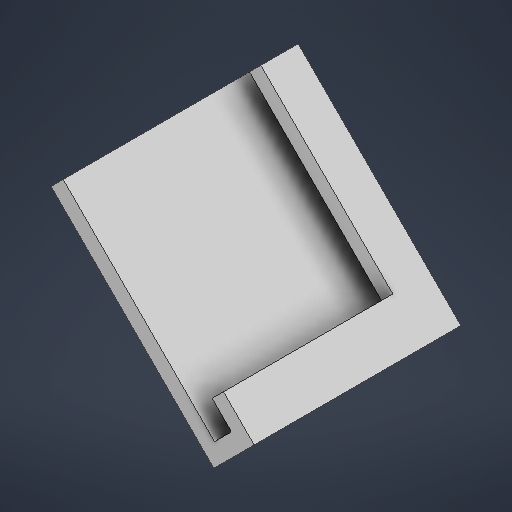
# Autodesk Inventor part: фанера
Saved by Autodesk Inventor 2025 (Build 290162000, 162)
## iProperties
Created: 2025-01-09
Part Number: фанера
Material: Типовые
Document SubType Name: Modeling
Designer: Phantom
Density: 1 g/cm^3
Appearance: По умолчанию
Author: Phantom
Autodesk Inventor part; units mm, degrees
ref_plane "YZ Plane" through (0, 0, 0) normal (1, 0, 0) x (0, 1, 0)
ref_plane "XZ Plane" through (0, 0, 0) normal (0, 1, 0) x (-1, 0, 0)
ref_plane "XY Plane" through (0, 0, 0) normal (0, 0, 1) x (1, 0, 0)
sketch "Эскиз1" plane through (0, 0, 0) normal (0, 0, 1) x (1, 0, 0)
  line L0 (0, 80) -> (80, 0)
  line L1 (2.2627, 82.2627) -> (82.2627, 2.2627)
  line L2 (0, 80) -> (2.2627, 82.2627)
  line L3 (80, 0) -> (82.2627, 2.2627)
  point P0 (0, 0)
  dimension "d2" = 3.2
  constraints: 8 end point, 2 perpendicular, 1 parallel
  measures "d2" distance between parallel lines of L0 L1
extrude "Выдавливание1" add sketch "Эскиз1" along normal blind 38.75
sketch "Эскиз2" plane through (0, 0, 0) normal (0, 0, -1) x (-1, 0, 0)
  line L0 (0, 80) -> (-80, 0) projected
  line L1 (-55, 25) -> (-55, -25)
  line L2 (-80, 0) -> (-55, 0)
  line L3 (-55, 8) -> (-60, 8)
  line L4 (-60, 8) -> (-60, 33)
  circle A0 centre (-60, 12) radius 2
  circle A1 centre (-60, 5) radius 2
  point P0 (0, 0)
  dimension "d5" = 4
  constraints: 8 end point, 3 point on line, 2 centre point, 1 horizontal, 1 midpoint, 1 perpendicular, 1 vertical
  measures "d5" diameter of A0
extrude "Выдавливание2" add sketch "Эскиз2" against normal blind 3 contours L1 L3 L4 A0 L0 | L4 A0 L3 L1 L2 L0
sketch "Эскиз3" plane through (2.2627, 82.2627, 0) normal (0.7071068, 0.7071068, 0) x (-0.7071068, 0.7071068, 0)
  line L0 (-113.1371, 0) -> (-95.4594, 0) projected
  line L1 (0, 38.75) -> (-113.1371, 38.75) projected
  line L2 (-113.1371, 0) -> (-110.1371, 0)
  line L3 (-110.1371, 0) -> (-110.1371, 38.75)
  line L4 (-110.1371, 38.75) -> (-113.1371, 38.75)
  line L5 (-113.1371, 38.75) -> (-113.1371, 0)
  point P0 (-56.5685, 0)
  point P1 (-113.1371, 38.75)
  dimension "d8" = 3
  constraints: 8 end point, 2 parallel, 1 horizontal, 1 perpendicular, 1 point on line
  measures "d8" distance of L4.end L3.end
extrude "Выдавливание3" add sketch "Эскиз3" along normal blind 4.5
sketch "Эскиз4" plane through (5.4447, 85.4447, 0) normal (0.7071068, 0.7071068, 0) x (0, 0, 1)
  line L0 (0, 113.1371) -> (3, 113.1371) projected
  line L1 (0, 0) -> (38.75, 0) projected
  line L2 (0, 113.1371) -> (7, 113.1371)
  line L3 (7, 113.1371) -> (7, 0)
  line L4 (7, 0) -> (0, 0)
  line L5 (0, 0) -> (0, 113.1371)
  line L6 (38.75, 0) -> (38.75, 113.1371) projected
  line L7 (7, 113.1371) -> (38.75, 113.1371)
  line L8 (38.75, 113.1371) -> (38.75, 105)
  line L9 (38.75, 105) -> (7, 105)
  line L10 (7, 105) -> (7, 113.1371)
  point P0 (0, 56.5685)
  point P1 (38.75, 113.1371)
  point P2 (7, 105)
  constraints: 16 end point, 4 parallel, 2 horizontal, 2 perpendicular, 2 point on line
extrude "Выдавливание4" add sketch "Эскиз4" along normal blind 3 contours L0 L2 L3 L1 L5 | L7 L6 L9 L3
sketch "Эскиз5" plane through (0, 0, 0) normal (0, 0, -1) x (-1, 0, 0)
  line L0 (-80.1414, 4.3841) -> (-2.2627, 82.2627) projected
  circle A0 centre (-60, 12) radius 2 projected
  circle A1 centre (-60, 5) radius 2 projected
  line L1 (0, 80) -> (-55, 25) projected
  line L2 (-2.2627, 82.2627) -> (0, 80) projected
  line L3 (-80.1414, 4.3841) -> (-2.2627, 82.2627) projected
  line L4 (-80.1414, 4.3841) -> (-83.3234, 7.566) projected
  line L5 (-83.3234, 7.566) -> (-5.4447, 85.4447) projected
  line L6 (-5.4447, 85.4447) -> (-7.566, 87.566) projected
  line L7 (-87.566, 7.566) -> (-7.566, 87.566) projected
  line L8 (-80, 0) -> (-87.566, 7.566) projected
  line L9 (-80, 0) -> (-55, 0) projected
  line L10 (-55, 0) -> (-55, 25) projected
  line L11 (-5.4447, 85.4447) -> (-2.2627, 82.2627)
  line L12 (-83.3234, 7.566) -> (-5.4447, 85.4447) projected
  point P0 (0, 0)
  point P1 (-2.2627, 82.2627)
  constraints: 2 end point, 1 perpendicular
extrude "Выдавливание5" add sketch "Эскиз5" against normal blind 3 contours L4 L5 L11 L0
sketch "Эскиз6" plane through (7.566, 87.566, 0) normal (0.7071068, 0.7071068, 0) x (-0.7071068, 0.7071068, 0)
  line L0 (0, 0) -> (-77.7817, 0) projected
  line L1 (-110.1371, 38.75) -> (0, 38.75) projected
  line L2 (0, 0) -> (-70, 0)
  line L3 (-70, 0) -> (-70, 38.75)
  line L4 (-70, 38.75) -> (0, 38.75)
  line L5 (0, 38.75) -> (0, 0)
  point P0 (-56.5685, 0)
  point P1 (0, 38.75)
  constraints: 8 end point, 2 parallel, 1 horizontal, 1 perpendicular, 1 point on line
extrude "Выдавливание6" cut sketch "Эскиз6" against normal through all
